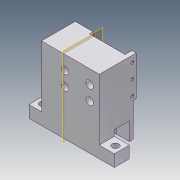
# Autodesk Inventor part: J005333
Saved by Autodesk Inventor 2015 SP1 (Build 190203100, 203)
## iProperties
Created: 2015-08-10
Material: ALUMINUM, 6061-T651
Vendor: HHMI: JRC - ID&F
Document SubType Name: Modeling
Designer: ARNOLDJ
Density: 2.7 g/cm^3
Appearance: Metal-AL-6061 (Machined)
Part Number: J005333
Project: P-201804
Description: MBS VSR GUIDE RAIL
RuleStatus: InUse
AfterDocSave0: file://Part Number Cleaner
LAB/DEPT: SVOBODA (LAB)
REQUESTING SCIENTIST: SOFRONIEW, NICK
SURFACE ROUGHNESS: 63 Ra
DESIGN DEPARTMENT: HHMI: JRC - ID&F
SPECIAL FINISH: ANODIZE PER MIL-A-8625F, TYPE II, CLASS 2 (BLACK)
ALTERED ITEM PART NUMBER: N/A
ALTERED ITEM VENDOR: N/A
ALTERED ITEM DESCRIPTION: N/A
Revision Number: -
Autodesk Inventor part; units mm, degrees
note: some values were not read from the file. Chosen so that the rebuilt part matches the saved one: direction of "Hole3".
ref_plane "XZ Plane" through (0, 0, 0) normal (0, 1, 0) x (-1, 0, 0)
ref_plane "XY Plane" through (0, 0, 0) normal (0, 0, 1) x (1, 0, 0)
sketch "Sketch1" plane through (0, 0, 0) normal (0, 0, 1) x (1, 0, 0)
  line L0 (29.845, -31.115) -> (-29.845, -31.115)
  line L1 (-29.845, -31.115) -> (-29.845, 31.115)
  line L2 (-29.845, 31.115) -> (29.845, 31.115)
  line L3 (29.845, 31.115) -> (29.845, -31.115)
  line L4 (29.845, -31.115) -> (-29.845, 31.115) construction
  line L5 (-29.845, -31.115) -> (29.845, 31.115) construction
  point P0 (0, 0)
  dimension "d0" = 59.69
  dimension "d1" = 62.23
  constraints: 12 end point, 2 midpoint, 2 parallel, 1 horizontal, 1 perpendicular
  measures "d0" distance of L1.end L2.end
  measures "d1" distance of L0.end L1.end
extrude "Extrusion1" add sketch "Sketch1" along normal blind 28.575
sketch "Sketch2" plane through (-29.845, 31.115, 0) normal (0, 1, 0) x (1, 0, 0)
  line L0 (0, 0) -> (59.69, 0) projected
  line L1 (59.69, 0) -> (59.69, -28.575) projected
  line L2 (56.134, 0) -> (25.88, 0)
  line L3 (25.88, 0) -> (25.88, -3.175)
  line L4 (25.88, -3.175) -> (56.134, -3.175)
  line L5 (59.69, 0) -> (0, 0) projected
  line L6 (56.134, 0) -> (56.134, -3.175)
  point P0 (29.845, 0)
  dimension "d4" = 3.175
  dimension "d5" = 30.254
  dimension "d52" = 3.556
  constraints: 8 end point, 2 perpendicular, 1 horizontal, 1 parallel, 1 point on line
  measures "d4" distance of L2.end L3.end
  measures "d5" distance of L3.end L4.end
  measures "d52" distance between parallel lines of L6 L1
extrude "Extrusion2" cut sketch "Sketch2" against normal blind 38.735
sketch "Sketch3" plane through (0, 0, 0) normal (0, 0, 1) x (1, 0, 0)
  point P0 (0, 0)
sketch "Sketch4" plane through (0, 0, 28.575) normal (0, 0, 1) x (1, 0, 0)
  line L0 (0.535, 7.4422) -> (21.535, 7.4422) construction
  line L1 (21.535, 7.4422) -> (21.535, 19.4422) construction
  line L2 (21.535, 19.4422) -> (0.535, 19.4422) construction
  line L3 (0.535, 19.4422) -> (0.535, 7.4422) construction
  line L4 (-29.845, -31.115) -> (29.845, -31.115) projected
  line L5 (-3.965, 31.115) -> (-3.965, -7.62) projected
  point P0 (0, 0)
  dimension "d8" = 21
  dimension "d9" = 12
  dimension "d10" = 38.5572
  dimension "d11" = 4.5
  constraints: 8 end point, 4 coincident, 2 parallel, 1 horizontal, 1 perpendicular
  measures "d8" distance of L1.end L2.end
  measures "d9" distance of L0.end L1.end
  measures "d10" distance between parallel lines of L4 L0
  measures "d11" distance between parallel lines of L3 L5
hole "Hole1" at (0.535, 19.4422, 28.575) at (0.535, 7.4422, 28.575) at (21.535, 7.4422, 28.575) at (21.535, 19.4422, 28.575) direction (0, 0, -1) diameter 2.8702 end through all counterbore diameter 6.35 counterbore depth 21.209
fillet "Fillet1" radius 3.175 2 edges at (-3.965, -7.62, 1.5875) (26.289, -7.62, 1.5875)
sketch "Sketch5" plane through (29.845, -31.115, 28.575) normal (1, 0, 0) x (0, 0, -1)
  line L0 (0, 0) -> (12.7, 0)
  line L1 (12.7, 0) -> (12.7, 10.16)
  line L2 (12.7, 10.16) -> (0, 10.16)
  line L3 (0, 10.16) -> (0, 0)
  point P0 (28.575, 31.115)
  dimension "d20" = 12.7
  dimension "d21" = 10.16
  constraints: 8 end point, 2 parallel, 1 horizontal, 1 perpendicular
  measures "d20" distance of L1.end L2.end
  measures "d21" distance of L0.end L1.end
extrude "Extrusion3" add sketch "Sketch5" along normal blind 12.7
sketch "Sketch6" plane through (-29.845, -31.115, 0) normal (0, -1, 0) x (1, 0, 0)
  line L0 (29.845, 34.29) -> (29.845, -5.715) projected
  line L1 (0, 28.575) -> (72.39, 28.575) projected
  line L2 (72.39, 28.575) -> (72.39, 15.875) projected
  line L3 (0, 0) -> (0, 28.575) projected
  point P0 (67.0052, 22.225)
  point P1 (5.4102, 22.225)
  point P2 (5.4102, 5.715)
  dimension "d39" = 6.35
  dimension "d40" = 37.1602
  dimension "d41" = 16.51
  dimension "d42" = 61.595
  dimension "d67" = 5.3848
  dimension "d68" = 5.4102
  constraints: 1 horizontal alignment, 1 vertical alignment
  measures "d39" distance from line of L1 point (67.005, 22.225)
  measures "d40" distance from line of point (67.005, 22.225) L0
  measures "d41" distance of point (5.41, 5.715) point (5.41, 22.225)
  measures "d42" distance of point (5.41, 22.225) point (67.005, 22.225)
  measures "d67" distance from line of point (67.005, 22.225) L2
  measures "d68" distance from line of point (5.41, 22.225) L3
hole "Hole2" at (37.1602, -31.115, 22.225) at (-24.4348, -31.115, 22.225) at (-24.4348, -31.115, 5.715) direction (0, 1, 0) diameter 5.7912 depth 12.7 tip angle 118
sketch "Sketch7" plane through (0, 0, 0) normal (0, 0, 1) x (1, 0, 0)
  line L0 (29.845, -20.955) -> (42.545, -20.955) projected
  line L1 (-29.845, 31.115) -> (-29.845, -31.115) projected
  line L2 (-29.845, -31.115) -> (42.545, -31.115) projected
  line L3 (29.845, 31.115) -> (-29.845, 31.115) projected
  line L4 (-29.845, -20.955) -> (-19.2024, -20.955)
  line L5 (-19.2024, -20.955) -> (-19.2024, 31.115)
  line L6 (-19.2024, 31.115) -> (-29.845, 31.115)
  line L7 (-29.845, 31.115) -> (-29.845, -20.955)
  point P0 (0, 0)
  dimension "d35" = 10.6426
  dimension "d36" = 10.16
  dimension "d43" = 0
  constraints: 8 end point, 2 parallel, 1 horizontal, 1 perpendicular, 1 point on line
  measures "d35" distance of L5.end L6.end
  measures "d36" distance between parallel lines of L4 L2
  measures "d43" distance between parallel lines of L6 L3
extrude "Extrusion4" cut sketch "Sketch7" along normal up to next
sketch "Sketch8" plane through (-29.845, -20.955, 28.575) normal (0, 1, 0) x (1, 0, 0)
  circle A0 centre (5.4102, 22.86) radius 2.8956 projected
  point P0 (29.845, 28.575)
sketch "Sketch9" plane through (-29.845, -31.115, 0) normal (0, -1, 0) x (1, 0, 0)
  line L0 (59.69, 15.875) -> (72.39, 15.875) projected
  line L1 (59.69, 0) -> (59.69, 15.875) projected
  line L2 (59.69, 0) -> (59.69, 28.575) construction
  line L3 (59.69, 15.875) -> (45.72, 15.875)
  line L4 (45.72, 15.875) -> (45.72, 3.175)
  line L5 (45.72, 3.175) -> (59.69, 3.175)
  line L6 (59.69, 3.175) -> (59.69, 15.875)
  line L7 (59.69, 0) -> (0, 0) construction
  point P0 (29.845, 0)
  point P1 (59.69, 3.175)
  dimension "d44" = 13.97
  dimension "d46" = 0
  dimension "d48" = 3.175
  constraints: 8 end point, 2 parallel, 1 horizontal, 1 perpendicular, 1 point on line
  measures "d44" distance of L3.start L3.end
  measures "d46" distance between parallel lines of L3 L0
  measures "d48" distance between parallel lines of L7 L5
extrude "Extrusion5" cut sketch "Sketch9" against normal blind 15.24
fillet "Fillet2" radius 3.175 2 edges at (15.875, -23.495, 3.175) (15.875, -23.495, 15.875)
sketch "Sketch10" plane through (0, 0, 0) normal (0, 0, -1) x (-1, 0, 0)
  line L0 (-29.845, 31.115) -> (-29.845, -31.115) projected
  line L1 (-26.289, 31.115) -> (-29.845, 31.115) projected
  line L2 (-26.289, -4.445) -> (-26.289, 31.115) projected
  line L3 (-29.845, 31.115) -> (-26.289, 31.115)
  line L4 (-26.289, 31.115) -> (-26.289, -2.54)
  line L5 (-26.289, -2.54) -> (-29.845, -2.54)
  line L6 (-29.845, -2.54) -> (-29.845, 31.115)
  point P0 (0, 0)
  dimension "d53" = 33.655
  constraints: 8 end point, 2 parallel, 1 horizontal, 1 perpendicular, 1 point on line
  measures "d53" distance between parallel lines of L1 L5
extrude "Extrusion6" add sketch "Sketch10" along normal blind 2.54
sketch "Sketch11" plane through (29.845, -20.955, 28.575) normal (1, 0, 0) x (0, 0, -1)
  line L0 (0, 52.07) -> (31.115, 52.07) projected
  line L1 (31.115, 52.07) -> (31.115, 18.415) projected
  point P0 (28.575, 20.955)
  point P1 (27.94, 46.6852)
  point P2 (27.94, 22.098)
  point P3 (27.94, 34.3916)
  dimension "d56" = 3.175
  dimension "d57" = 5.3848
  dimension "d58" = 24.5872
  dimension "d66" = 12.2936
  constraints: 2 vertical alignment
  measures "d56" distance from line of point (27.94, 46.685) L1
  measures "d57" distance from line of point (27.94, 46.685) L0
  measures "d58" distance of point (27.94, 46.685) point (27.94, 22.098)
  measures "d66" distance of point (27.94, 22.098) point (27.94, 34.392)
hole "Hole3" at (29.845, 25.7302, 0.635) at (29.845, 1.143, 0.635) at (29.845, 13.4366, 0.635) direction (-1, 0, 0) diameter 2.4638 end up to surface
equation "\"d66\" = 0.5 * d58"
body "Solid1"
